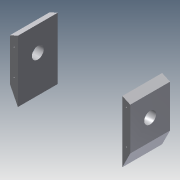
# Autodesk Inventor part: predni strana
Saved by Autodesk Inventor 2013 (Build 170138000, 138)
## iProperties
Created: 2012-08-22
Part Number: predni strana
Material: Generic
Document SubType Name: Modeling
Designer: idle-rug
Density: 1 g/cm^3
Author: idle-rug
Autodesk Inventor part; units mm, degrees
ref_plane "YZ Plane" through (0, 0, 0) normal (1, 0, 0) x (0, 1, 0)
ref_plane "XZ Plane" through (0, 0, 0) normal (0, 1, 0) x (-1, 0, 0)
ref_plane "XY Plane" through (0, 0, 0) normal (0, 0, 1) x (1, 0, 0)
sketch "Sketch1" plane through (0, 0, 0) normal (0, 1, 0) x (-1, 0, 0)
  line L0 (65.5, 26.5) -> (75.5, 26.5)
  line L1 (75.5, 26.5) -> (75.5, -26.5)
  line L2 (75.5, -26.5) -> (65.5, -26.5)
  line L3 (65.5, -46.5) -> (75.5, -26.5)
  line L4 (-65.5, 26.5) -> (-75.5, 26.5)
  line L5 (-75.5, 26.5) -> (-75.5, -26.5)
  line L6 (-75.5, -26.5) -> (-65.5, -26.5)
  line L7 (-65.5, -46.5) -> (-75.5, -26.5)
  line L8 (75.5, 26.5) -> (65.5, 30.9444)
  line L9 (-75.5, 26.5) -> (-65.5, 30.9444)
  line L10 (65.5, 30.9444) -> (65.5, -46.5)
  line L11 (-65.5, -46.5) -> (-65.5, 30.9444)
  dimension "d3" = 10
  dimension "d4" = 53
  dimension "d8" = 10
  dimension "d9" = 53
  constraints: 24 end point, 1 parallel, 1 perpendicular
  measures "d3" distance of L0.start L0.end
  measures "d4" distance of L0.end L1.end
  measures "d8" distance of L4.start L4.end
  measures "d9" distance of L4.end L5.end
extrude "Extrusion1" add sketch "Sketch1" along normal blind 50
sketch "Sketch4" plane through (75.5, 0, 26.5) normal (1, 0, 0) x (0, 0, -1)
  circle A0 centre (26.5, 25) radius 7.5
  dimension "d15" = 15
  constraints: 1 centre point
  measures "d15" diameter of A0
hole "Hole1" at (75.5, 25, 0) direction (-1, 0, 0) diameter 15 depth 151
sketch "Sketch5" plane through (0, 0, 0) normal (0, -1, 0) x (1, 0, 0)
  circle A0 centre (-70.5, 16.5) radius 2.9966
  point P0 (0, 0)
  constraints: 1 centre point
hole "Hole2" at (-70.5, 0, 16.5) direction (0, 1, 0) diameter 2 depth 50
sketch "Sketch6" plane through (0, 0, 0) normal (0, -1, 0) x (1, 0, 0)
  circle A0 centre (-70.5, -16.5) radius 3.2107
  point P0 (0, 0)
  constraints: 1 centre point
hole "Hole3" at (-70.5, 0, -16.5) direction (0, 1, 0) diameter 2 depth 50
sketch "Sketch8" plane through (0, 0, 0) normal (0, -1, 0) x (1, 0, 0)
  circle A0 centre (70.5, -21.5) radius 2.6808
  circle A1 centre (70.5, 21.5) radius 3.2604
  point P0 (0, 0)
  constraints: 2 centre point
hole "Hole4" at (70.5, 0, 21.5) at (70.5, 0, -21.5) direction (0, 1, 0) diameter 2 depth 50
body "Solid1"
